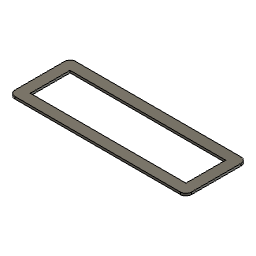
baseNUC v0 (Autodesk Fusion 360 design; units mm, degrees)
Autodesk Fusion 360 part; units mm, degrees
sketch "Sketch1" plane through (0, 0, 0) normal (0, 1, 0) x (1, 0, 0)
  line L0 (70.5, 18) -> (-70.5, 18)
  line L1 (-70.5, 18) -> (-70.5, -18)
  line L2 (-70.5, -18) -> (70.5, -18)
  line L3 (70.5, -18) -> (70.5, 18)
  line L4 (70.5, 18) -> (-70.5, -18) construction
  line L5 (-70.5, 18) -> (70.5, -18) construction
  line L6 (80, 27.5) -> (-80, 27.5)
  line L7 (-80, 27.5) -> (-80, -27.5)
  line L8 (-80, -27.5) -> (80, -27.5)
  line L9 (80, -27.5) -> (80, 27.5)
  line L10 (80, 27.5) -> (-80, -27.5) construction
  line L11 (-80, 27.5) -> (80, -27.5) construction
  dimension "d1" = 141
  dimension "d2" = 36
  dimension "d3" = 160
  dimension "d4" = 55
  constraint horizontal L0
  constraint perpendicular L0 L1
  constraint parallel L0 L2
  constraint parallel L1 L3
  constraint coincident L4 origin
  constraint coincident L5 origin
  constraint horizontal L6
  constraint perpendicular L6 L7
  constraint parallel L6 L8
  constraint parallel L7 L9
  constraint coincident L10 origin
  constraint coincident L11 origin
  measures "d1" distance of L1.end L2.end
  measures "d2" distance of L0.end L1.end
  measures "d3" distance of L7.end L8.end
  measures "d4" distance of L6.end L7.end
extrude "Extrude1" add sketch "Sketch1" along normal blind 2
fillet "Fillet1" radius 5 1 edges at (-80, 1, 27.5)
fillet "Fillet2" radius 5 1 edges at (80, 1, 27.5)
fillet "Fillet3" radius 5 1 edges at (80, 1, -27.5)
fillet "Fillet4" radius 5 1 edges at (-80, 1, -27.5)
